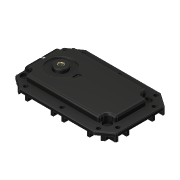
# Autodesk Inventor part: Depan
Saved by Autodesk Inventor 2019 (Build 230136000, 136)
## iProperties
Created: 2021-08-24
Part Number: Depan
Material: Generic
Document SubType Name: Modeling
Designer: user
Density: 1 g/cm^3
Appearance: Glossy - Black
Author: user
Autodesk Inventor part; units mm, degrees
ref_plane "YZ Plane" through (0, 0, 0) normal (1, 0, 0) x (0, 1, 0)
ref_plane "XZ Plane" through (0, 0, 0) normal (0, 1, 0) x (-1, 0, 0)
ref_plane "XY Plane" through (0, 0, 0) normal (0, 0, 1) x (1, 0, 0)
sketch "Sketch1" plane through (0, 0, 0) normal (0, 1, 0) x (-1, 0, 0)
  line L0 (30.55, -20.1) -> (-30.55, -20.1)
  line L1 (-30.55, -20.1) -> (-30.55, 20.1)
  line L2 (-30.55, 20.1) -> (30.55, 20.1)
  line L3 (30.55, 20.1) -> (30.55, -20.1)
  line L4 (30.55, -20.1) -> (-30.55, 20.1) construction
  line L5 (-30.55, -20.1) -> (30.55, 20.1) construction
  circle A0 centre (17.55, 0) radius 1.25
  circle A1 centre (17.55, 0) radius 14
  line L6 (-24.95, -14.5) -> (30.55, -14.5)
  line L7 (30.55, -14.5) -> (30.55, 14.5)
  line L8 (30.55, 14.5) -> (-24.95, 14.5)
  line L9 (-24.95, 14.5) -> (-24.95, -14.5)
  line L10 (-24.95, -14.5) -> (30.55, 14.5) construction
  line L11 (30.55, -14.5) -> (-24.95, 14.5) construction
  circle A2 centre (21.55, 17.3) radius 1.25
  circle A3 centre (21.55, -17.3) radius 1.25
  circle A4 centre (-0.45, 17.3) radius 1.25
  circle A5 centre (-0.45, -17.3) radius 1.25
  circle A6 centre (-22.45, 17.3) radius 1.25
  circle A7 centre (-22.45, -17.3) radius 1.25
  circle A8 centre (-27.75, -11) radius 1.25
  circle A9 centre (-27.75, 11) radius 1.25
  line L12 (30.55, 14.5) -> (22.55, 20.1)
  line L13 (-30.55, 14.5) -> (-22.55, 20.1)
  line L14 (30.55, -14.5) -> (22.55, -20.1)
  line L15 (-30.55, -14.5) -> (-22.55, -20.1)
  line L16 (-30.55, -14.5) -> (24.95, -14.5)
  circle A10 centre (-17.55, 0) radius 1.25
  line L17 (24.95, 14.5) -> (-30.55, 14.5)
  line L18 (-30.55, 9.5) -> (-30.55, -9.5)
  line L19 (19.95, 14.5) -> (-25.55, 14.5)
  line L20 (-25.55, -14.5) -> (19.95, -14.5)
  circle A11 centre (-17.55, 0) radius 1.25
  circle A12 centre (-17.55, 0) radius 1.25
  circle A13 centre (-22.45, 12) radius 2.5
  circle A14 centre (-22.45, -12) radius 2.5
  circle A15 centre (27.05, -12) radius 2.5
  circle A16 centre (27.05, 12) radius 2.5
  line L21 (-24.95, -12) -> (-24.95, -14.5)
  line L22 (-24.95, -14.5) -> (-22.45, -14.5)
  line L23 (-24.95, 14.5) -> (-22.45, 14.5)
  line L24 (-24.95, 14.5) -> (-24.95, 12)
  line L25 (-22.45, -14.5) -> (-24.95, -14.5)
  line L26 (-24.95, -14.5) -> (-24.95, -12)
  arc A17 (-24.95, -12) -> (-22.45, -14.5) centre (-22.45, -12) ccw
  line L27 (-24.95, 12) -> (-24.95, 14.5)
  line L28 (-24.95, 14.5) -> (-22.45, 14.5)
  arc A18 (-22.45, 14.5) -> (-24.95, 12) centre (-22.45, 12) ccw
  point P0 (0, 0)
  point P1 (2.8, 0)
  point P2 (30.55, 0)
  point P3 (0, 0)
  point P4 (-30.55, 0)
  point P5 (-2.8, 0)
  point P6 (0, 0)
  point P7 (0, 0)
  point P8 (-30.55, 0)
  dimension "d0" = 61.1
  dimension "d1" = 40.2
  dimension "d2" = 2.5
  dimension "d3" = 13
  dimension "d4" = 28
  dimension "d5" = 55.5
  dimension "d9" = 4
  dimension "d10" = 2.8
  dimension "d13" = 34.6
  dimension "d16" = 22
  dimension "d20" = 2.8
  dimension "d23" = 22
  dimension "d24" = 11
  dimension "d25" = 8
  dimension "d100" = 2.5
  dimension "d101" = 29
  dimension "d102" = 5
  dimension "d103" = 5
  dimension "d104" = 24
  constraints: 58 end point, 19 centre point, 10 point on line, 8 point on circle, 6 midpoint, 6 parallel, 6 tangent, 4 collinear, 4 perpendicular, 3 horizontal, 2 coincident, 1 concentric, 1 vertical, 1 vertical alignment, 10 other
  measures "d0" distance of L1.end L2.end
  measures "d1" distance of L0.end L1.end
  measures "d2" diameter of A0
  measures "d3" distance from line of L3 A0.centre
  measures "d4" diameter of A1
  measures "d5" distance of L8.end L7.end
  measures "d9" horizontal distance of A2.centre A0.centre
  measures "d10" distance from line of L2 A2.centre
  measures "d13" distance of A2.centre A3.centre
  measures "d16" distance of A2.centre A4.centre
  measures "d20" distance from line of L1 A8.centre
  measures "d23" distance of A9.centre A8.centre
  measures "d24" vertical distance of A8.centre point (0, 0)
  measures "d25" distance of L2.end L12.end
  measures "d100" diameter of A10
  measures "d101" distance of L16.start L17.end
  measures "d102" diameter of A13
  measures "d103" diameter of A14
  measures "d104" distance of A13.centre A14.centre
extrude "Extrusion10" add sketch "Sketch1" against normal blind 4.6 contours L0 L15 L16 L6 L14 | L6 A15 A1 L3 | A1 A15 A16 L3 | L6 A14 L9 A13 L8 A16 A1 A15 | A15 A1 | L1 L17 L9 L16 | A1 A16 L8 L3 | A1 A15 | L8 L17 L13 L2 L12 | A16 A1 | A1 A16 | L9 A14 L6 | A14 | L9 L8 A13 | A13 | A10
sketch "Sketch20" plane through (0, 0, 0) normal (0, 1, 0) x (1, 0, 0)
  circle A0 centre (-27.05, -12) radius 2.5
  circle A1 centre (-27.05, 12) radius 2.5
  circle A2 centre (-17.55, 0) radius 1.25
  circle A3 centre (22.45, -12) radius 2.5
  circle A4 centre (22.45, 12) radius 2.5
  line L0 (-30.55, -14.5) -> (-30.55, 14.5)
  line L1 (24.95, 14.5) -> (-30.55, 14.5)
  line L2 (-30.55, 14.5) -> (-30.55, -14.5)
  line L3 (-30.55, -14.5) -> (24.95, -14.5)
  line L4 (24.95, -14.5) -> (24.95, 14.5)
  line L5 (-22.55, -20.1) -> (-30.55, -14.5)
  line L6 (-30.55, -14.5) -> (-24.55, -14.5)
  line L7 (-24.55, -14.5) -> (-24.55, -12)
  line L8 (-27.05, -9.5) -> (-30.55, -9.5)
  line L9 (-30.55, -9.5) -> (-30.55, -14.5)
  line L10 (-30.55, 14.5) -> (-24.55, 14.5)
  line L11 (-24.55, 14.5) -> (-24.55, 12)
  line L12 (-27.05, 9.5) -> (-30.55, 9.5)
  line L13 (-30.55, 9.5) -> (-30.55, 14.5)
  line L14 (24.95, 14.5) -> (19.95, 14.5)
  line L15 (19.95, 14.5) -> (19.95, 12)
  line L16 (22.45, 9.5) -> (24.95, 9.5)
  line L17 (24.95, 9.5) -> (24.95, 14.5)
  line L18 (24.95, -14.5) -> (19.95, -14.5)
  line L19 (19.95, -14.5) -> (19.95, -12)
  line L20 (22.45, -9.5) -> (24.95, -9.5)
  line L21 (24.95, -9.5) -> (24.95, -14.5)
  line L22 (-30.55, 14.5) -> (-24.55, 14.5)
  line L23 (-24.55, 14.5) -> (-24.55, 12)
  line L24 (-27.05, 9.5) -> (-30.55, 9.5)
  line L25 (-30.55, 9.5) -> (-30.55, 14.5)
  line L26 (-30.55, -14.5) -> (-24.55, -14.5)
  line L27 (-24.55, -14.5) -> (-24.55, -12)
  line L28 (-27.05, -9.5) -> (-30.55, -9.5)
  line L29 (-30.55, -9.5) -> (-30.55, -14.5)
  point P0 (0, 0)
  point P1 (0, 0)
  constraints: 60 end point, 14 parallel, 8 point on circle, 7 horizontal, 7 perpendicular, 5 centre point
extrude "Extrusion18" add sketch "Sketch20" along normal blind 3.5 contours A0 L8 L0 L12 A1 L11 L1 L15 A4 L16 L4 L20 A3 L19 L3 L7
sketch "Sketch21" plane through (0, 0, 0) normal (0, 1, 0) x (1, 0, 0)
  circle A0 centre (-27.05, -12) radius 2.5
  circle A1 centre (-27.05, 12) radius 2.5
  circle A2 centre (-17.55, 0) radius 1.25
  circle A3 centre (22.45, -12) radius 2.5
  circle A4 centre (22.45, 12) radius 2.5
  line L0 (-30.55, -14.5) -> (-30.55, 14.5)
  line L1 (24.95, 14.5) -> (-30.55, 14.5)
  line L2 (-30.55, 14.5) -> (-30.55, -14.5)
  line L3 (-30.55, -14.5) -> (24.95, -14.5)
  line L4 (24.95, -14.5) -> (24.95, 14.5)
  line L5 (-22.55, -20.1) -> (-30.55, -14.5)
  line L6 (-30.55, -14.5) -> (-24.55, -14.5)
  line L7 (-24.55, -14.5) -> (-24.55, -12)
  line L8 (-27.05, -9.5) -> (-30.55, -9.5)
  line L9 (-30.55, -9.5) -> (-30.55, -14.5)
  line L10 (-30.55, 14.5) -> (-24.55, 14.5)
  line L11 (-24.55, 14.5) -> (-24.55, 12)
  line L12 (-27.05, 9.5) -> (-30.55, 9.5)
  line L13 (-30.55, 9.5) -> (-30.55, 14.5)
  line L14 (24.95, 14.5) -> (19.95, 14.5)
  line L15 (19.95, 14.5) -> (19.95, 12)
  line L16 (22.45, 9.5) -> (24.95, 9.5)
  line L17 (24.95, 9.5) -> (24.95, 14.5)
  line L18 (24.95, -14.5) -> (19.95, -14.5)
  line L19 (19.95, -14.5) -> (19.95, -12)
  line L20 (22.45, -9.5) -> (24.95, -9.5)
  line L21 (24.95, -9.5) -> (24.95, -14.5)
  line L22 (-30.55, 14.5) -> (-24.55, 14.5)
  line L23 (-24.55, 14.5) -> (-24.55, 12)
  line L24 (-27.05, 9.5) -> (-30.55, 9.5)
  line L25 (-30.55, 9.5) -> (-30.55, 14.5)
  line L26 (-30.55, -14.5) -> (-24.55, -14.5)
  line L27 (-24.55, -14.5) -> (-24.55, -12)
  line L28 (-27.05, -9.5) -> (-30.55, -9.5)
  line L29 (-30.55, -9.5) -> (-30.55, -14.5)
  point P0 (0, 0)
  point P1 (0, 0)
  point P2 (0, 0)
  constraints: 60 end point, 14 parallel, 8 point on circle, 7 horizontal, 7 perpendicular, 5 centre point
extrude "Extrusion19" cut sketch "Sketch21" against normal blind 2 contours A0 | A3 | A1 | A4
sketch "Sketch22" plane through (0, 3.5, 0) normal (0, 1, 0) x (1, 0, 0)
  circle A0 centre (-17.55, 0) radius 1.25 projected
  circle A1 centre (-17.55, 0) radius 7.5
  line L0 (-6.55, -2) -> (-9.05, -2)
  line L1 (-9.05, -2) -> (-9.05, 2)
  line L2 (-9.05, 2) -> (-6.55, 2)
  line L3 (-6.55, 2) -> (-6.55, -2)
  line L4 (-6.55, -2) -> (-9.05, 2) construction
  line L5 (-9.05, -2) -> (-6.55, 2) construction
  point P0 (0, 0)
  point P1 (-7.8, 0)
  dimension "d168" = 15
  dimension "d169" = 2.5
  dimension "d170" = 4
  dimension "d171" = 1
  constraints: 12 end point, 2 midpoint, 2 parallel, 1 centre point, 1 coincident, 1 horizontal, 1 perpendicular
  measures "d168" diameter of A1
  measures "d169" distance of L1.end L2.end
  measures "d170" distance of L0.end L1.end
  measures "d171" distance edge to line of A1 L1
extrude "Extrusion20" cut sketch "Sketch22" against normal blind 1 contours A0 | A1 | L0 L1 L2 L3
sketch "Sketch23" plane through (-17.55, 2.5, 0) normal (0, 1, 0) x (1, 0, 0)
  circle A0 centre (0, 0) radius 1.25 projected
  circle A1 centre (0, 0) radius 4
  circle A2 centre (0, 0) radius 1.25
  point P0 (17.55, 0)
  dimension "d174" = 8
  constraints: 2 centre point, 2 coincident
  measures "d174" diameter of A1
extrude "Extrusion21" add sketch "Sketch23" along normal blind 2.5
sketch "Sketch19" plane through (0, -4.6, 0) normal (0, -1, 0) x (1, 0, 0)
  line L0 (-22.2348, -20.1) -> (22.2348, -20.1)
  circle A0 centre (-21.55, -17.3) radius 1.25
  line L1 (-21.55, -14.4132) -> (-19.05, -15.8566)
  line L2 (-19.05, -15.8566) -> (-19.05, -18.7434)
  line L3 (-19.05, -18.7434) -> (-21.55, -20.1868)
  line L4 (-21.55, -20.1868) -> (-24.05, -18.7434)
  line L5 (-24.05, -18.7434) -> (-24.05, -15.8566)
  line L6 (-24.05, -15.8566) -> (-21.55, -14.4132)
  line L7 (-17.55, -19.6094) -> (-17.55, -14.9906)
  line L8 (-17.55, -14.9906) -> (-21.55, -12.6812)
  line L9 (-21.55, -12.6812) -> (-25.55, -14.9906)
  line L10 (-25.55, -14.9906) -> (-25.55, -19.6094)
  line L11 (-25.55, -19.6094) -> (-21.55, -21.9188)
  line L12 (-21.55, -21.9188) -> (-17.55, -19.6094)
  circle A1 centre (27.75, -11) radius 1.25
  line L13 (24.8632, -11) -> (26.3066, -8.5)
  line L14 (26.3066, -8.5) -> (29.1934, -8.5)
  line L15 (29.1934, -8.5) -> (30.6368, -11)
  line L16 (30.6368, -11) -> (29.1934, -13.5)
  line L17 (29.1934, -13.5) -> (26.3066, -13.5)
  line L18 (26.3066, -13.5) -> (24.8632, -11)
  line L19 (23.1312, -11) -> (25.4406, -7)
  line L20 (25.4406, -7) -> (30.0594, -7)
  line L21 (30.0594, -7) -> (32.3688, -11)
  line L22 (32.3688, -11) -> (30.0594, -15)
  line L23 (30.0594, -15) -> (25.4406, -15)
  line L24 (25.4406, -15) -> (23.1312, -11)
  line L25 (0.45, -12.6812) -> (-3.55, -14.9906)
  line L26 (-2.05, -15.8566) -> (0.45, -14.4132)
  line L27 (4.45, -14.9906) -> (0.45, -12.6812)
  line L28 (0.45, -14.4132) -> (2.95, -15.8566)
  line L29 (-2.05, -18.7434) -> (-2.05, -15.8566)
  line L30 (-3.55, -14.9906) -> (-3.55, -19.6094)
  line L31 (-3.55, -19.6094) -> (0.45, -21.9188)
  line L32 (0.45, -20.1868) -> (-2.05, -18.7434)
  line L33 (2.95, -15.8566) -> (2.95, -18.7434)
  line L34 (4.45, -19.6094) -> (4.45, -14.9906)
  line L35 (2.95, -18.7434) -> (0.45, -20.1868)
  line L36 (0.45, -21.9188) -> (4.45, -19.6094)
  line L37 (22.45, -12.6812) -> (18.45, -14.9906)
  line L38 (19.95, -15.8566) -> (22.45, -14.4132)
  line L39 (26.45, -14.9906) -> (22.45, -12.6812)
  line L40 (22.45, -14.4132) -> (24.95, -15.8566)
  line L41 (19.95, -18.7434) -> (19.95, -15.8566)
  line L42 (18.45, -14.9906) -> (18.45, -19.6094)
  line L43 (18.45, -19.6094) -> (22.45, -21.9188)
  line L44 (22.45, -20.1868) -> (19.95, -18.7434)
  line L45 (24.95, -15.8566) -> (24.95, -18.7434)
  line L46 (26.45, -19.6094) -> (26.45, -14.9906)
  line L47 (24.95, -18.7434) -> (22.45, -20.1868)
  line L48 (22.45, -21.9188) -> (26.45, -19.6094)
  line L49 (30.55, 13.9793) -> (30.55, -13.9793)
  line L50 (30.55, 0) -> (-30.55, 0)
  line L51 (-30.55, 13.9793) -> (-30.55, -13.9793)
  line L52 (22.2348, -20.1) -> (-22.2348, -20.1)
  line L53 (4.45, -14.9906) -> (18.45, -14.9906)
  line L54 (18.45, -14.9906) -> (18.45, -20.1)
  line L55 (18.45, -20.1) -> (4.45, -20.1)
  line L56 (4.45, -20.1) -> (4.45, -14.9906)
  line L57 (-3.55, -14.9906) -> (-17.55, -14.9906)
  line L58 (-17.55, -14.9906) -> (-17.55, -20.1)
  line L59 (-17.55, -20.1) -> (-3.55, -20.1)
  line L60 (-3.55, -20.1) -> (-3.55, -14.9906)
  line L61 (-22.8082, -19.9192) -> (-29.9795, -14.8994)
  line L62 (-25.55, -14.9906) -> (-25.55, -18)
  line L63 (-25.55, -18) -> (-29.8789, -14.9698)
  line L64 (-24.05, -18.7434) -> (-19.05, -18.7434)
  line L65 (-19.05, -18.7434) -> (-19.05, -20.1)
  line L66 (-19.05, -20.1) -> (-24.05, -20.1)
  line L67 (-24.05, -20.1) -> (-24.05, -18.7434)
  line L68 (2.95, -18.7434) -> (-2.05, -18.7434)
  line L69 (-2.05, -18.7434) -> (-2.05, -20.1)
  line L70 (-2.05, -20.1) -> (2.95, -20.1)
  line L71 (2.95, -20.1) -> (2.95, -18.7434)
  line L72 (19.95, -18.7434) -> (24.95, -18.7434)
  line L73 (24.95, -18.7434) -> (24.95, -20.1)
  line L74 (24.95, -20.1) -> (19.95, -20.1)
  line L75 (19.95, -20.1) -> (19.95, -18.7434)
  line L76 (29.1934, -13.5) -> (30.55, -13.5)
  line L77 (30.55, -13.5) -> (30.55, -8.5)
  line L78 (30.55, -8.5) -> (29.1934, -8.5)
  line L79 (29.1934, -8.5) -> (29.1934, -13.5)
  line L80 (26.45, -15) -> (30.2607, -15)
  line L81 (30.2607, -15) -> (30.2607, -17.4093)
  line L82 (30.2607, -17.4093) -> (26.45, -17.4093)
  line L83 (26.45, -17.4093) -> (26.45, -15)
  line L84 (25.4406, -7) -> (30.55, -7)
  line L85 (30.55, -7) -> (30.55, 0)
  line L86 (30.55, 0) -> (25.4406, 0)
  line L87 (25.4406, 0) -> (25.4406, -7)
  line L88 (23.95, -14.5) -> (-28.55, -14.5)
  line L89 (18.45, -20.1) -> (4.45, -20.1)
  line L90 (4.45, -20.1) -> (4.45, -14.5)
  line L91 (4.45, -14.5) -> (18.45, -14.5)
  line L92 (18.45, -14.5) -> (18.45, -20.1)
  line L93 (-17.55, -20.1) -> (-3.55, -20.1)
  line L94 (-3.55, -20.1) -> (-3.55, -14.5)
  line L95 (-3.55, -14.5) -> (-17.55, -14.5)
  line L96 (-17.55, -14.5) -> (-17.55, -20.1)
  line L97 (-25.55, -18) -> (-25.55, -14.5)
  line L98 (-29.55, -14.5) -> (23.95, -14.5)
  line L99 (-25.55, -14.5) -> (-29.55, -14.5)
  line L100 (-29.55, -14.5) -> (-29.8789, -14.9698)
  line L101 (-29.8789, -14.9698) -> (-25.55, -18)
  line L102 (-30.55, -11.25) -> (-30.55, 11.25)
  circle A2 centre (-21.55, 17.3) radius 1.25
  line L103 (-21.55, 14.4132) -> (-19.05, 15.8566)
  line L104 (-19.05, 15.8566) -> (-19.05, 18.7434)
  line L105 (-19.05, 18.7434) -> (-21.55, 20.1868)
  line L106 (-17.55, 19.6094) -> (-17.55, 14.9906)
  line L107 (-17.55, 14.9906) -> (-21.55, 12.6812)
  line L108 (-24.05, 15.8566) -> (-21.55, 14.4132)
  line L109 (-24.05, 18.7434) -> (-24.05, 15.8566)
  line L110 (-21.55, 20.1868) -> (-24.05, 18.7434)
  line L111 (-21.55, 12.6812) -> (-25.55, 14.9906)
  line L112 (-25.55, 14.9906) -> (-25.55, 19.6094)
  circle A3 centre (27.75, 11) radius 1.25
  line L113 (24.8632, 11) -> (26.3066, 8.5)
  line L114 (25.4406, 15) -> (23.1312, 11)
  line L115 (26.3066, 13.5) -> (24.8632, 11)
  line L116 (29.1934, 13.5) -> (26.3066, 13.5)
  line L117 (30.0594, 15) -> (25.4406, 15)
  line L118 (26.3066, 8.5) -> (29.1934, 8.5)
  line L119 (25.4406, 7) -> (30.0594, 7)
  line L120 (23.1312, 11) -> (25.4406, 7)
  line L121 (-22.2348, 20.1) -> (22.2348, 20.1)
  line L122 (23.95, 14.5) -> (-28.55, 14.5)
  line L123 (-29.55, 14.5) -> (23.95, 14.5)
  line L124 (22.2348, 20.1) -> (-22.2348, 20.1)
  line L125 (-3.55, 14.9906) -> (-3.55, 19.6094)
  line L126 (-2.05, 18.7434) -> (-2.05, 15.8566)
  line L127 (-2.05, 18.7434) -> (-2.05, 20.1)
  line L128 (-2.05, 15.8566) -> (0.45, 14.4132)
  line L129 (0.45, 20.1868) -> (-2.05, 18.7434)
  line L130 (2.95, 18.7434) -> (0.45, 20.1868)
  line L131 (2.95, 18.7434) -> (-2.05, 18.7434)
  line L132 (2.95, 15.8566) -> (2.95, 18.7434)
  line L133 (4.45, 14.9906) -> (0.45, 12.6812)
  line L134 (0.45, 12.6812) -> (-3.55, 14.9906)
  line L135 (0.45, 14.4132) -> (2.95, 15.8566)
  line L136 (-3.55, 20.1) -> (-3.55, 14.5)
  line L137 (-3.55, 20.1) -> (-3.55, 14.9906)
  line L138 (-17.55, 20.1) -> (-3.55, 20.1)
  line L139 (-17.55, 20.1) -> (-3.55, 20.1)
  line L140 (-17.55, 14.9906) -> (-17.55, 20.1)
  line L141 (-3.55, 14.9906) -> (-17.55, 14.9906)
  line L142 (-3.55, 14.5) -> (-17.55, 14.5)
  line L143 (4.45, 14.9906) -> (18.45, 14.9906)
  line L144 (18.45, 20.1) -> (4.45, 20.1)
  line L145 (4.45, 19.6094) -> (4.45, 14.9906)
  line L146 (4.45, 20.1) -> (4.45, 14.9906)
  line L147 (2.95, 20.1) -> (2.95, 18.7434)
  line L148 (30.0594, 7) -> (32.3688, 11)
  line L149 (32.3688, 11) -> (30.0594, 15)
  line L150 (18.45, 14.9906) -> (18.45, 20.1)
  line L151 (18.45, 14.9906) -> (18.45, 19.6094)
  line L152 (19.95, 18.7434) -> (19.95, 15.8566)
  line L153 (19.95, 15.8566) -> (22.45, 14.4132)
  line L154 (22.45, 12.6812) -> (18.45, 14.9906)
  line L155 (24.95, 15.8566) -> (24.95, 18.7434)
  line L156 (22.45, 14.4132) -> (24.95, 15.8566)
  line L157 (26.45, 19.6094) -> (26.45, 14.9906)
  line L158 (26.45, 14.9906) -> (22.45, 12.6812)
  line L159 (-2.05, 20.1) -> (2.95, 20.1)
  line L160 (0.45, 21.9188) -> (4.45, 19.6094)
  line L161 (-3.55, 19.6094) -> (0.45, 21.9188)
  line L162 (18.45, 19.6094) -> (22.45, 21.9188)
  line L163 (22.45, 20.1868) -> (19.95, 18.7434)
  line L164 (24.95, 18.7434) -> (22.45, 20.1868)
  line L165 (22.45, 21.9188) -> (26.45, 19.6094)
  line L166 (26.45, 15) -> (30.2607, 15)
  line L167 (26.45, 17.4093) -> (26.45, 15)
  line L168 (30.2607, 15) -> (30.2607, 17.4093)
  line L169 (24.95, 18.7434) -> (24.95, 20.1)
  line L170 (19.95, 18.7434) -> (24.95, 18.7434)
  line L171 (24.95, 20.1) -> (19.95, 20.1)
  line L172 (19.95, 20.1) -> (19.95, 18.7434)
  line L173 (18.45, 14.5) -> (18.45, 20.1)
  line L174 (4.45, 14.5) -> (18.45, 14.5)
  line L175 (4.45, 20.1) -> (4.45, 14.5)
  line L176 (18.45, 20.1) -> (4.45, 20.1)
  line L177 (30.2607, 17.4093) -> (26.45, 17.4093)
  line L178 (29.1934, 8.5) -> (30.6368, 11)
  line L179 (30.6368, 11) -> (29.1934, 13.5)
  line L180 (29.1934, 13.5) -> (30.55, 13.5)
  line L181 (30.55, 13.5) -> (30.55, 8.5)
  line L182 (30.55, 8.5) -> (29.1934, 8.5)
  line L183 (25.4406, 7) -> (30.55, 7)
  line L184 (29.1934, 8.5) -> (29.1934, 13.5)
  line L185 (-25.55, 19.6094) -> (-21.55, 21.9188)
  line L186 (-21.55, 21.9188) -> (-17.55, 19.6094)
  line L187 (-17.55, 14.5) -> (-17.55, 20.1)
  line L188 (-19.05, 18.7434) -> (-19.05, 20.1)
  line L189 (-19.05, 20.1) -> (-24.05, 20.1)
  line L190 (-24.05, 20.1) -> (-24.05, 18.7434)
  line L191 (-25.55, 14.9906) -> (-25.55, 18)
  line L192 (-25.55, 18) -> (-25.55, 14.5)
  line L193 (-25.55, 14.5) -> (-29.55, 14.5)
  line L194 (-29.55, 14.5) -> (-29.8789, 14.9698)
  line L195 (-25.55, 18) -> (-29.8789, 14.9698)
  line L196 (-29.8789, 14.9698) -> (-25.55, 18)
  line L197 (-22.8082, 19.9192) -> (-29.9795, 14.8994)
  line L198 (-24.05, 18.7434) -> (-19.05, 18.7434)
  line L199 (30.55, -13.9793) -> (30.55, 13.9793)
  line L200 (25.4406, 0) -> (25.4406, 7)
  line L201 (25.4406, 7) -> (30.55, 7)
  line L202 (30.55, 7) -> (30.55, 0)
  line L203 (30.55, 0) -> (25.4406, 0)
  line L204 (25.4406, 0) -> (25.4406, 7)
  line L205 (-30.55, -14.5) -> (-30.55, 14.5) projected
  line L206 (-29.55, 14.5) -> (-30.55, 14.5)
  line L207 (-30.55, 14.5) -> (-29.8789, 14.9698)
  line L208 (-29.8789, 14.9698) -> (-29.55, 14.5)
  line L209 (-30.55, -14.5) -> (-22.55, -20.1) projected
  line L210 (-30.55, -14.5) -> (-29.55, -14.5)
  line L211 (-29.55, -14.5) -> (-29.8789, -14.9698)
  line L212 (-29.8789, -14.9698) -> (-30.55, -14.5)
  line L213 (-25.55, -18) -> (-30.55, -14.5)
  line L214 (-30.55, -14.5) -> (-25.55, -14.5)
  line L215 (-25.55, -14.5) -> (-25.55, -18)
  line L216 (-25.55, -18) -> (-25.55, -14.9906)
  line L217 (-25.55, -14.9906) -> (-21.55, -12.6812)
  line L218 (-21.55, -12.6812) -> (-17.55, -14.9906)
  line L219 (-17.55, -14.9906) -> (-17.55, -20.1)
  point P0 (0, 0)
  point P1 (0, 0)
  point P2 (0.45, -17.3)
  point P3 (0.45, -17.3)
  point P4 (-0.2348, -20.1)
  point P5 (22.45, -17.3)
  point P6 (22.45, -17.3)
  point P7 (21.7652, -20.1)
  point P8 (0.45, 17.3)
  point P9 (0.45, 17.3)
  point P10 (21.7652, 20.1)
  point P11 (22.45, 17.3)
  point P12 (22.45, 17.3)
  point P13 (-0.2348, 20.1)
  point P14 (-30.55, 9.5)
  dimension "d155" = 5
  dimension "d156" = 1.5
  dimension "d157" = 5
  dimension "d158" = 1.5
  dimension "d159" = 22
  dimension "d160" = 22.5
  constraints: 436 end point, 99 symmetric about line, 30 point on line, 24 parallel, 17 perpendicular, 14 horizontal, 8 coincident, 6 collinear, 4 centre point, 2 midpoint, 92 other
  measures "d155" distance between parallel lines of L5 L2
  measures "d156" distance between parallel lines of L2 L7
  measures "d157" distance between parallel lines of L14 L17
  measures "d158" distance between parallel lines of L18 L24
  measures "d159" distance of L9.end L25.end
  measures "d160" distance of L102.start L102.end
extrude "Extrusion17" cut sketch "Sketch19" against normal blind 2.6 contours L58 L7 L57 L30 L60 L0 | L0 L3 L65 | L96 L88 L94 L57 | L69 L32 L0 | L3 L4 L0 | L0 L4 L64 L3 | L64 L5 L6 L88 L1 L2 | L32 L68 L35 L0 | L0 L35 L32 | L29 L26 L88 L28 L33 L68 | L0 L66 L209 L61 L67 L4 | L61 L100 L98 L88 L97 L10 | L88 L6 L1 | L35 L71 L0 | L56 L34 L53 L42 L54 L0 | L26 L28 L88 | L61 L209 L66 L67 | L61 L209 L210 L100 | L90 L88 L92 L53 | L75 L44 L74 L0 | L72 L47 L74 L44 | L41 L38 L88 L40 L45 L72 | L38 L40 L88 | L74 L47 L44 | L73 L74 L47 | L46 L23 L80 L81 L82 | L200 L119 L183 L49 L50 | L50 L49 L84 L20 L87 | L207 L197 L194 L206 | L194 L195 L112 L192 L122 L123 | L117 L157 L177 L168 L166 | L153 L152 L170 L155 L156 L122 | L122 L156 L153 | L122 L175 L143 L173 | L143 L145 L146 L121 L150 | L190 L189 L121 L110 | L122 L103 L108 | L108 L109 L198 L104 L103 L122 | L110 L121 L105 L198 | L172 L121 L171 L163 | L163 L171 L164 L170 | L110 L105 L121 | L105 L121 L188 | L164 L171 L169 | L163 L164 L171 | L135 L128 L122 | L122 L128 L126 L131 L132 L135 | L106 L140 L121 L136 L125 L141 | L141 L136 L122 L187 | L147 L130 L121 | L131 L129 L121 L130 | L121 L129 L130 | L127 L121 L129 | L13 L14 L79 L17 L18 | L78 L49 L15 | L15 L49 L16 L79 | L16 L49 L76 | L15 L16 L49 | L49 L179 L180 | L179 L178 L49 | L49 L178 L184 L179 | L184 L118 L113 L115 L116 | L49 L182 L178
fillet "Fillet5" radius 3.5 1 edges at (-30.55, 3.5, 0)
fillet "Fillet6" radius 1 31 edges at (-2.3, 3.5, -14.5) (-29.5249, 2.4749, -9.5) (-24.55, 3.5, -13.25) (-25.2822, 3.5, -10.2322) (-24.55, 1.75, -14.5) (24.95, 1.75, -9.5) (20.6822, 3.5, -10.2322) (19.95, 3.5, -13.25) (23.7, 3.5, -9.5) (19.95, 1.75, -14.5) (24.95, 3.5, 0) (24.95, 1.75, 9.5) (23.7, 3.5, 9.5) (19.95, 3.5, 13.25) (20.6822, 3.5, 10.2322) (19.95, 1.75, 14.5) (-2.3, 3.5, 14.5) (-24.55, 1.75, 14.5) (-24.55, 3.5, 13.25) (-29.5249, 2.4749, 9.5) (-25.2822, 3.5, 10.2322) (-30.55, -3.3, -14.5) (-30.55, -1, -14.5) (-30.55, -3.3, 14.5) (-30.55, -1, 14.5) (-22.55, -1, 20.1) (-22.55, -1, -20.1) (30.55, -2.3, -14.5) (22.55, -1, -20.1) (30.55, -2.3, 14.5) (22.55, -1, 20.1)
fillet "Fillet7" radius 0.5 22 edges at (22.5354, 0, 20.0537) (26.4659, 0, 17.3589) (30.437, 0, 14.4412) (30.55, 0, 0) (30.437, 0, -14.4412) (26.4659, 0, -17.3589) (22.5354, 0, -20.0537) (0, 0, -20.1) (-22.5354, 0, -20.0537) (-26.4659, 0, -17.3589) (-30.437, 0, -14.4412) (-30.55, 0, -9) (-30.55, 0, -11.7397) (-22.5354, 0, 20.0537) (-26.4659, 0, 17.3589) (-30.437, 0, 14.4412) (-30.55, 0, 9) (-30.55, 0, 11.7397) (0, 0, 20.1) (-18.8, 5, 0) (-21.55, 5, 0) (-25.05, 3.5, 0)
sketch "Sketch24" plane through (0, 0, 0) normal (0, 0, 1) x (1, 0, 0)
  line L0 (-27.05, 2.5) -> (-27.05, 3.5) projected
  line L1 (-27.05, 3.5) -> (-27.05, -2)
  line L2 (-25.55, -2) -> (-30.1235, -2) projected
  line L3 (-30.55, -0.5) -> (-30.55, -2) projected
  line L4 (-27.05, -2) -> (-30.55, -2)
  line L5 (-30.1235, -2) -> (-30.55, -2) projected
  line L6 (-30.55, -2) -> (-30.55, 0)
  arc A0 (-27.05, 3.5) -> (-30.55, 0) centre (-27.05, 0) ccw
  arc A1 (-27.05, 3.5) -> (-30.55, 0) centre (-27.05, 0) ccw projected
  arc A2 (-27.05, 3.5) -> (-30.55, 0) centre (-27.05, 0) ccw
  point P0 (0, 0)
  constraints: 6 end point, 4 point on circle, 2 centre point, 2 vertical, 1 horizontal, 1 point on line
extrude "Extrusion22" cut sketch "Sketch24" along normal mid plane 2
sketch "Sketch25" plane through (0, 0, 0) normal (0, 0, 1) x (1, 0, 0)
  line L0 (-27.05, 2.5) -> (-27.05, 3.5)
  line L1 (-27.05, 3.5) -> (-27.05, -2)
  line L2 (-27.05, -2) -> (-30.1235, -2)
  line L3 (-27.05, -2) -> (-30.55, -2)
  line L4 (-30.1235, -2) -> (-30.55, -2)
  arc A0 (-27.05, 3.5) -> (-30.55, 0) centre (-27.05, 0) ccw projected
  line L5 (-30.55, -2) -> (-30.55, 0) projected
  line L6 (-27.05, -2) -> (-30.55, -2) projected
  line L7 (-27.05, 3.5) -> (-27.05, -2) projected
  arc A1 (-27.05, 3.2) -> (-30.25, 0) centre (-27.05, 0) ccw
  line L8 (-30.25, 0) -> (-30.25, -2)
  line L9 (-30.55, -2) -> (-29.55, -2) projected
  line L10 (-30.25, -2) -> (-27.05, -2)
  line L11 (-27.05, -2) -> (-27.05, 3.2)
  line L12 (-27.05, 2.5) -> (-27.05, 3.5) projected
  point P0 (0, 0)
  point P1 (0, 0)
  dimension "d185" = 3.2
  dimension "d186" = 3.2
  constraints: 16 end point, 2 point on circle, 2 vertical, 1 centre point, 1 collinear, 1 horizontal, 1 perpendicular, 1 point on line
  measures "d185" radius of A1
  measures "d186" distance between parallel lines of L11 L8
extrude "Extrusion23" add sketch "Sketch25" along normal mid plane 1.8 contours L1 L2 L3 L8 A1 L0
thread "Thread1" size "M3x0.5" class "6H" standard "ANSI Metric M Profile" full length
body "Solid1"
body "Solid3"
